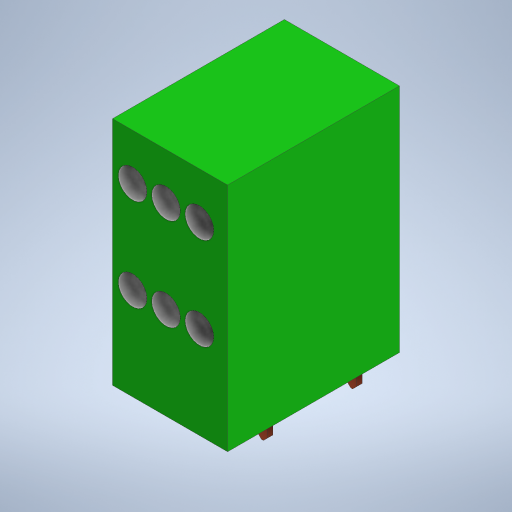
# Autodesk Inventor part: KF207RH
Saved by Autodesk Inventor 2024 (Build 280153000, 153)
## iProperties
Created: 2023-05-20
Part Number: KF207RH
Material: Generic
Document SubType Name: Modeling
Designer: Torban Peterson
Density: 1 g/cm^3
Appearance: Default
Author: Torban Peterson
Autodesk Inventor part; units mm, degrees
ref_plane "YZ Plane" through (0, 0, 0) normal (1, 0, 0) x (0, 1, 0)
ref_plane "XZ Plane" through (0, 0, 0) normal (0, 1, 0) x (-1, 0, 0)
ref_plane "XY Plane" through (0, 0, 0) normal (0, 0, 1) x (1, 0, 0)
sketch "Sketch2" plane through (0, 0, 0) normal (0, 0, 1) x (1, 0, 0)
  line L0 (0, 0) -> (12.05, 0)
  line L1 (12.05, 0) -> (12.05, 24.2)
  line L2 (12.05, 24.2) -> (0, 24.2)
  line L3 (0, 24.2) -> (0, 0)
  dimension "d0" = 12.05
  dimension "d1" = 24.2
  constraints: 8 end point, 2 parallel, 1 horizontal, 1 perpendicular
  measures "d0" distance of L1.end L2.end
  measures "d1" distance between parallel lines of L0 L2
extrude "Extrusion1" add sketch "Sketch2" against normal blind 18
sketch "Sketch3" plane through (0, 0, 0) normal (0, -1, 0) x (1, 0, 0)
  line L0 (2.1, -6.9) -> (5.6, -6.9) construction
  line L1 (5.6, -6.9) -> (5.6, -16.25) construction
  line L2 (5.6, -16.25) -> (2.1, -16.25) construction
  line L3 (2.1, -16.25) -> (2.1, -6.9) construction
  line L4 (12.05, -18) -> (0, -18) construction
  line L5 (0, 0) -> (0, -18) construction
  line L6 (0, 0) -> (12.05, 0) construction
  line L7 (5.6, -6.9) -> (9.1, -6.9) construction
  line L8 (9.1, -6.9) -> (9.1, -16.25) construction
  line L9 (9.1, -16.25) -> (5.6, -16.25) construction
  line L10 (5.6, -16.25) -> (5.6, -6.9) construction
  line L11 (1.6, -6.6) -> (2.6, -6.6)
  line L12 (2.6, -6.6) -> (2.6, -7.2)
  line L13 (2.6, -7.2) -> (1.6, -7.2)
  line L14 (1.6, -7.2) -> (1.6, -6.6)
  line L15 (1.6, -6.6) -> (2.6, -7.2) construction
  line L16 (2.6, -6.6) -> (1.6, -7.2) construction
  line L17 (5.1, -6.6) -> (6.1, -6.6)
  line L18 (6.1, -6.6) -> (6.1, -7.2)
  line L19 (6.1, -7.2) -> (5.1, -7.2)
  line L20 (5.1, -7.2) -> (5.1, -6.6)
  line L21 (8.6, -6.6) -> (9.6, -6.6)
  line L22 (9.6, -6.6) -> (9.6, -7.2)
  line L23 (9.6, -7.2) -> (8.6, -7.2)
  line L24 (8.6, -7.2) -> (8.6, -6.6)
  line L25 (1.6, -15.95) -> (2.6, -15.95)
  line L26 (2.6, -15.95) -> (2.6, -16.55)
  line L27 (2.6, -16.55) -> (1.6, -16.55)
  line L28 (1.6, -16.55) -> (1.6, -15.95)
  line L29 (5.1, -15.95) -> (6.1, -15.95)
  line L30 (6.1, -15.95) -> (6.1, -16.55)
  line L31 (6.1, -16.55) -> (5.1, -16.55)
  line L32 (5.1, -16.55) -> (5.1, -15.95)
  line L33 (8.6, -15.95) -> (9.6, -15.95)
  line L34 (9.6, -15.95) -> (9.6, -16.55)
  line L35 (9.6, -16.55) -> (8.6, -16.55)
  line L36 (8.6, -16.55) -> (8.6, -15.95)
  dimension "d5" = 2.1
  dimension "d6" = 6.9
  dimension "d7" = 9.35
  dimension "d8" = 3.5
  dimension "d11" = 3.5
  dimension "d16" = 1
  dimension "d17" = 0.6
  dimension "d20" = 3.5
  dimension "d23" = 9.35
  constraints: 68 end point, 5 coincident, 4 horizontal, 4 parallel, 3 collinear, 2 midpoint, 2 perpendicular, 1 vertical, 45 other
  measures "d5" distance between parallel lines of L5 L3
  measures "d6" distance between parallel lines of L0 L6
  measures "d7" distance between parallel lines of L2 L0
  measures "d8" distance between parallel lines of L1 L3
  measures "d11" distance of L0.start L7.start
  measures "d16" distance between parallel lines of L12 L14
  measures "d17" distance between parallel lines of L13 L11
  measures "d20" distance of L11.start L17.start
  measures "d23" distance of L11.start L25.start
extrude "Extrusion2" add sketch "Sketch3" along normal blind 3.7 separate body
chamfer "Chamfer1" distance 0.4 angle 45 12 edges at (2.6, -3.7, -6.9) (1.6, -3.7, -6.9) (5.1, -3.7, -6.9) (6.1, -3.7, -6.9) (8.6, -3.7, -6.9) (9.6, -3.7, -6.9) (8.6, -3.7, -16.25) (9.6, -3.7, -16.25) (6.1, -3.7, -16.25) (5.1, -3.7, -16.25) (2.6, -3.7, -16.25) (1.6, -3.7, -16.25)
sketch "Sketch4" plane through (0, 0, 0) normal (0, 0, 1) x (1, 0, 0)
  line L0 (2.2, -3.7) -> (2, -3.7) construction
  line L1 (5.7, -3.7) -> (5.5, -3.7) construction
  line L2 (9.2, -3.7) -> (9, -3.7) construction
  line L3 (12.05, 0) -> (12.05, 24.2) construction
  line L4 (12.05, 24.2) -> (0, 24.2) construction
  line L5 (0, 24.2) -> (0, 0) construction
  line L6 (0, 0) -> (12.05, 0) construction
  line L7 (0, 19.36) -> (12.05, 19.36) construction
  line L8 (0, 14.52) -> (12.05, 14.52) construction
  line L9 (0, 9.68) -> (12.05, 9.68) construction
  line L10 (0, 4.84) -> (12.05, 4.84) construction
  line L11 (2.1, -3.7) -> (2.1, 19.36) construction
  line L12 (5.6, -3.7) -> (5.6, 19.36) construction
  line L13 (9.1, -3.7) -> (9.1, 19.36) construction
  point P0 (6.025, 19.36)
  point P1 (6.025, 14.52)
  point P2 (6.025, 9.68)
  point P3 (6.025, 4.84)
  point P4 (2.1, 9.68)
  point P5 (5.6, 9.68)
  point P6 (9.1, 9.68)
  dimension "d31" = 24.2
  dimension "d32" = 4.84
  dimension "d35" = 4.84
  constraints: 14 end point, 11 point on line, 4 midpoint, 4 perpendicular, 3 coincident, 1 vertical, 12 other
  measures "d31" distance between parallel lines of L6 L4
  measures "d32" distance from line of point (6.025, 19.36) L4
  measures "d35" distance of L7.start L8.start
hole "Hole1" at (2.1, 19.36, 0) at (2.1, 9.68, 0) at (5.6, 9.68, 0) at (5.6, 19.36, 0) at (9.1, 19.36, 0) at (9.1, 9.68, 0) direction (0, 0, -1) diameter 3 depth 8 tip angle 118 bodies 1
equation "\"d32\" = 0.2 * d31"
equation "\"d35\" = d32"
body "Solid1"
